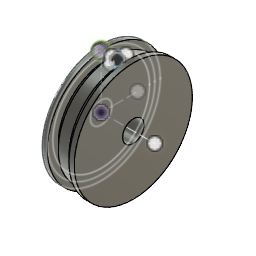
cylindrical_cam (Autodesk Fusion 360 design; units mm, degrees)
part number: 2026-06-02-07-36-12-330
Autodesk Fusion 360 part; units mm, degrees
note: some values were not read from the file. Chosen so that the rebuilt part matches the saved one: which bodies a step acts on; which face or edge a step refers to. Set by a fixed rule: which sketch regions a step uses.
sketch "Roata" plane through (0, 0, 0) normal (1, 0, 0) x (0, 1, 0)
  circle A0 centre (0, 0) radius 5
  circle A1 centre (0, 0) radius 25
  line L0 (0, 0) -> (0, 25) construction
  line L1 (0, 0) -> (17, 0) construction
  circle A2 centre (0, 0) radius 27.5
  circle A3 centre (0, 0) radius 22.5
  dimension "d1" = 10
  dimension "d2" = 50
  dimension "d7" = 55
  dimension "d42" = 45
  constraint coincident A0.centre A1.centre
  constraint concentric A0 A1
  constraint coincident A1 L0.end
  constraint vertical L0
  constraint horizontal L1
  measures "d1" diameter of A0
  measures "d2" diameter of A1
  measures "d7" diameter of A2
  measures "d42" diameter of A3
extrude "Extrude1" add sketch "Roata" along normal blind 2.5 contours A2 makes body 1
extrude "Extrude2" add sketch "Roata" along normal blind 2.5 from surface at 12.5 separate body contours A2 makes body 2
extrude "Extrude3" add sketch "Roata" along normal blind 15 contours A1 | A3 bodies 1 2
extrude "Extrude4" cut sketch "Roata" along normal blind 2.5 from surface at 2.5 contours A1 | A2 | A3 bodies 1 makes body 3 at (0, 19.879, -1.6146)
extrude "Extrude5" cut sketch "Roata" against normal blind 2.5 from surface at 12.5 contours A1 | A2 | A3 bodies 1 3 makes body 4 at (12.5, 19.879, -1.6146)
sketch "Ax" plane through (0, 0, 0) normal (0, 0, 1) x (1, 0, 0)
  line L0 (0, 0) -> (25, 0) construction
  constraint coincident L0.start origin
  constraint horizontal L0
ref_plane "WorkPlane1" through (6.315, 0, 25) normal (0, 0, 1) x (0, 1, 0)
sketch "fanta" plane through (0, 0, 25) normal (0, 0, 1) x (1, 0, 0)
  line L0 (5, 0) -> (9.501, 0) construction
  line L1 (0, 0) -> (0, -1) construction
  line L2 (7.5, -3) -> (7.5, 4.0716) construction
  line L3 (7.5, 0) -> (10, -2) construction
  line L4 (7.5, 0) -> (5, 2) construction
  line L5 (10, -0.3992) -> (4.9768, 3.6193)
  line L6 (10, -3.6008) -> (5, 0.3992)
  line L7 (5, 2) -> (5, 3.6008)
  line L8 (5, 2) -> (5, 0.3992)
  line L9 (10, -2) -> (10, -0.3992)
  line L10 (10, -2) -> (10, -3.3614)
  line L11 (10, -3.3614) -> (10, -3.6008)
  line L12 (10, -3.6008) -> (10.3027, -3.843)
  line L13 (10.3027, -3.843) -> (10.3027, -0.6414)
  line L14 (10, -0.3992) -> (10.3027, -0.6414)
  line L15 (5, 0.3992) -> (4.6861, 0.6503)
  line L16 (4.6861, 0.6503) -> (4.6861, 3.8519)
  line L17 (4.9768, 3.6193) -> (4.6861, 3.8519)
  point P0 (7.5, 0)
  dimension "d25" = 1
  dimension "d33" = 1.25
  constraint coincident L1.start origin
  constraint horizontal L0
  constraint perpendicular L0 L1
  constraint vertical L2
  constraint coincident P0 L3.start
  constraint parallel L3 L4
  constraint parallel L4 L5
  constraint vertical L7
  constraint perpendicular L0 L8
  constraint perpendicular L0 L9
  constraint parallel L9 L10
  constraint parallel L10 L11
  constraint coincident L5 L0.end
  constraint coincident L5 L7.end
  constraint parallel L6 L12
  constraint parallel L11 L13
  constraint parallel L5 L14
  constraint parallel L6 L15
  constraint parallel L8 L16
  constraint parallel L5 L17
  measures "d25" distance of L1.start L1.end
  measures "d33" distance of L3 L5
extrude "Extrude6" cut sketch "fanta" against normal blind 10 contours L5 L6 L7 L8 L9 L10 L11 bodies 1 3 4
extrude "Extrude8" cut sketch "fanta" along normal blind 10 from surface at -55 contours L5 L6 L7 L8 L9 L10 L11 bodies 1
extrude "Extrude10" add sketch "Roata" along normal blind 15 contours A3 bodies 1 3 4
equation "d10 = 10 mm + 2.5 mm"
named bodies: "Roata"
